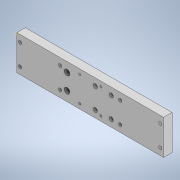
# Autodesk Inventor part: Head Adapter Plate
Saved by Autodesk Inventor 2020 (Build 240168000, 168)
## iProperties
Created: 2020-03-19
Part Number: Head Adapter Plate
Material: Generic
Document SubType Name: Modeling
Designer: DasNick
Density: 1 g/cm^3
Appearance: Default
Author: DasNick
Autodesk Inventor part; units mm, degrees
ref_plane "YZ Plane" through (0, 0, 0) normal (1, 0, 0) x (0, 1, 0)
ref_plane "XZ Plane" through (0, 0, 0) normal (0, 1, 0) x (-1, 0, 0)
ref_plane "XY Plane" through (0, 0, 0) normal (0, 0, 1) x (1, 0, 0)
sketch "Sketch1" plane through (0, 0, 0) normal (0, 0, 1) x (1, 0, 0)
  line L0 (13.4603, 15.4458) -> (13.4545, -36.9417)
  circle A0 centre (18.2181, -26.6234) radius 2.3812
  circle A1 centre (18.2217, 5.1266) radius 2.3812
  circle A2 centre (78.5467, 5.1199) radius 2.3812
  circle A3 centre (78.5431, -26.6301) radius 2.3812
  circle A4 centre (169.0306, -26.6401) radius 2.3812
  circle A5 centre (229.3556, -26.6468) radius 2.3812
  circle A6 centre (229.3592, 5.1032) radius 2.3812
  line L1 (234.1228, 15.4214) -> (234.117, -36.9661)
  circle A7 centre (169.0342, 5.1099) radius 2.3812
  line L2 (13.4545, -36.9417) -> (234.117, -36.9661)
  line L3 (234.1228, 15.4214) -> (13.4603, 15.4458)
  point P0 (3.3527, -2.3752)
  constraints: 8 centre point, 8 end point
extrude "Extrusion1" add sketch "Sketch1" along normal blind 12.7
sketch "Sketch3" plane through (0, 0, 0) normal (0, 0, -1) x (-1, 0, 0)
  line L0 (-234.117, -36.9661) -> (-234.1228, 15.4214) projected
  line L1 (-234.1199, -10.7723) -> (-13.4574, -10.7479)
  line L2 (-13.4603, 15.4458) -> (-13.4545, -36.9417) projected
  line L3 (-234.1228, 15.4214) -> (-13.4603, 15.4458) projected
  line L4 (-123.7915, 15.4336) -> (-123.7857, -36.9539)
  line L5 (-13.4545, -36.9417) -> (-234.117, -36.9661) projected
  circle A0 centre (-155.5369, -26.2636) radius 1.5
  circle A1 centre (-131.5369, -26.261) radius 1.5
  circle A2 centre (-155.5404, 4.7364) radius 1.5
  circle A3 centre (-131.5404, 4.739) radius 1.5
  point P0 (0, 0)
  dimension "d8" = 15.5
  dimension "d9" = 31.75
  dimension "d10" = 3
  dimension "d13" = 24
  dimension "d16" = 31
  constraints: 4 centre point, 4 end point, 3 midpoint, 10 other
  measures "d8" distance from line of L1 A0.centre
  measures "d9" distance from line of L4 A0.centre
  measures "d10" diameter of A0
  measures "d13" distance of A0.centre A1.centre
  measures "d16" distance of A0.centre A2.centre
extrude "Extrusion2" cut sketch "Sketch3" against normal blind 12.7 contours A0 | A1 | A2 | A3
sketch "Sketch4" plane through (0, 0, 0) normal (0, 0, -1) x (-1, 0, 0)
  circle A0 centre (-131.5369, -26.261) radius 1.5 projected
  circle A1 centre (-131.5369, -26.261) radius 3.175
  circle A2 centre (-155.5369, -26.2636) radius 1.5 projected
  circle A3 centre (-155.5369, -26.2636) radius 3.175
  circle A4 centre (-131.5404, 4.739) radius 1.5 projected
  circle A5 centre (-131.5404, 4.739) radius 3.175
  circle A6 centre (-155.5404, 4.7364) radius 1.5 projected
  circle A7 centre (-155.5404, 4.7364) radius 3.175
  point P0 (0, 0)
  dimension "d21" = 6.35
  dimension "d22" = 6.35
  dimension "d23" = 6.35
  dimension "d24" = 6.35
  constraints: 4 centre point, 4 coincident
  measures "d21" diameter of A1
  measures "d22" diameter of A3
  measures "d23" diameter of A5
  measures "d24" diameter of A7
extrude "Extrusion3" cut sketch "Sketch4" against normal blind 3.175
sketch "Sketch5" plane through (0, 0, 0) normal (0, 0, -1) x (-1, 0, 0)
  point P0 (0, 0)
sketch "Sketch6" plane through (0, 0, 0) normal (0, 0, -1) x (-1, 0, 0)
  point P0 (0, 0)
sketch "Sketch7" plane through (0, 0, 0) normal (0, 0, -1) x (-1, 0, 0)
  point P0 (0, 0)
sketch "Sketch8" plane through (0, 0, 0) normal (0, 0, -1) x (-1, 0, 0)
  circle A0 centre (-108.2333, 8.2916) radius 1.5875
  line L0 (-234.1228, 15.4214) -> (-13.4603, 15.4458) construction
  line L1 (-123.7915, 15.4336) -> (-123.7857, -36.9539) construction
  line L2 (-13.4545, -36.9417) -> (-234.117, -36.9661) construction
  line L3 (-234.117, -36.9661) -> (-234.1228, 15.4214) construction
  line L4 (-234.1199, -10.7723) -> (-13.4574, -10.7479) construction
  line L5 (-13.4603, 15.4458) -> (-13.4545, -36.9417) construction
  circle A1 centre (-108.229, -29.8084) radius 1.5875
  circle A2 centre (-139.9833, 8.2881) radius 1.5875
  circle A3 centre (-139.979, -29.8119) radius 1.5875
  point P0 (0, 0)
  dimension "d27" = 3.175
  dimension "d28" = 15.5575
  dimension "d31" = 38.1
  dimension "d34" = 31.75
  dimension "d37" = 19.05
  constraints: 4 centre point, 4 end point, 4 midpoint, 8 other
  measures "d27" diameter of A0
  measures "d28" distance from line of L1 A0.centre
  measures "d31" distance of A0.centre A1.centre
  measures "d34" distance of A0.centre A2.centre
  measures "d37" distance from line of L4 A0.centre
extrude "Extrusion4" cut sketch "Sketch8" against normal blind 25.4
sketch "Sketch9" plane through (0, 0, 12.7) normal (0, 0, 1) x (1, 0, 0)
  circle A0 centre (155.5369, -26.2636) radius 1.5 projected
  circle A1 centre (131.5369, -26.261) radius 1.5 projected
  circle A2 centre (155.5404, 4.7364) radius 1.5 projected
  circle A3 centre (131.5404, 4.739) radius 1.5 projected
  circle A4 centre (155.5369, -26.2636) radius 3.175
  circle A5 centre (131.5369, -26.261) radius 3.175
  circle A6 centre (131.5404, 4.739) radius 3.175
  circle A7 centre (155.5404, 4.7364) radius 3.175
  point P0 (0, 0)
  dimension "d40" = 6.35
  dimension "d41" = 6.35
  dimension "d42" = 6.35
  dimension "d43" = 6.35
  constraints: 4 centre point, 4 coincident
  measures "d40" diameter of A4
  measures "d41" diameter of A5
  measures "d42" diameter of A6
  measures "d43" diameter of A7
extrude "Extrusion5" cut sketch "Sketch9" against normal blind 3.175
sketch "Sketch10" plane through (0, 0, 0) normal (0, 0, -1) x (-1, 0, 0)
  circle A0 centre (-88.9984, 1.2723) radius 3.175 projected
  circle A1 centre (-88.9953, -22.4777) radius 3.175 projected
  circle A2 centre (-88.9953, -22.4777) radius 3.9688
  circle A3 centre (-88.9984, 1.2723) radius 3.9688
  point P0 (0, 0)
  dimension "d46" = 7.9375
  dimension "d47" = 7.9375
  constraints: 2 centre point, 2 coincident
  measures "d46" diameter of A2
  measures "d47" diameter of A3
extrude "Extrusion6" cut sketch "Sketch10" against normal blind 12.7 contours A0 | A1 | A2 | A3
fillet "Fillet1" radius 0.254 4 edges at (92.9672, 1.2723, 12.7) (92.9641, -22.4777, 12.7) (92.9641, -22.4777, 0) (92.9672, 1.2723, 0)
sketch "Sketch11" plane through (0, 0, 0) normal (0, 0, -1) x (-1, 0, 0)
  circle A0 centre (-88.9953, -22.4777) radius 3.9688
  circle A1 centre (-139.979, -29.8119) radius 1.5875
  circle A2 centre (-139.9833, 8.2881) radius 1.5875
  circle A3 centre (-108.229, -29.8084) radius 1.5875
  circle A4 centre (-108.2333, 8.2916) radius 1.5875
  circle A5 centre (-155.5404, 4.7364) radius 3.175
  circle A6 centre (-155.5369, -26.2636) radius 3.175
  circle A7 centre (-131.5404, 4.739) radius 3.175
  circle A8 centre (-131.5369, -26.261) radius 3.175
  line L0 (-13.4545, -36.9417) -> (-234.117, -36.9661)
  line L1 (-13.4603, 15.4458) -> (-13.4545, -36.9417)
  line L2 (-234.1228, 15.4214) -> (-13.4603, 15.4458)
  line L3 (-234.117, -36.9661) -> (-234.1228, 15.4214)
  circle A9 centre (-169.0342, 5.1099) radius 2.3812
  circle A10 centre (-229.3592, 5.1032) radius 2.3812
  circle A11 centre (-229.3556, -26.6468) radius 2.3812
  circle A12 centre (-169.0306, -26.6401) radius 2.3812
  circle A13 centre (-78.5431, -26.6301) radius 2.3812
  circle A14 centre (-78.5467, 5.1199) radius 2.3812
  circle A15 centre (-18.2217, 5.1266) radius 2.3812
  circle A16 centre (-18.2181, -26.6234) radius 2.3812
  circle A17 centre (-88.9984, 1.2723) radius 4.2227
  point P0 (0, 0)
  dimension "d51" = 10.3187
  dimension "d53" = 4.7625
  dimension "d54" = 220.6625
  dimension "d55" = 4.7625
  dimension "d56" = 65.0875
  dimension "d57" = 94.7738
  dimension "d58" = 118.0812
  dimension "d59" = 7.9375
  dimension "d60" = 126.5238
  dimension "d61" = 142.0813
  dimension "d62" = 155.575
  dimension "d63" = 215.9
  dimension "d64" = 14.4724
  dimension "d65" = 42.0688
  dimension "d66" = 7.1437
  dimension "d67" = 38.2224
  dimension "d68" = 10.6937
  dimension "d69" = 45.2437
  dimension "d70" = 41.6938
  dimension "d71" = 52.3875
  constraints: 35 centre point, 8 end point
  measures "d51" distance from line of L0 A16.centre
  measures "d53" diameter of A16
  measures "d54" distance of L0.start L0.end
  measures "d55" distance from line of A16.centre L1
  measures "d56" distance from line of A13.centre L1
  measures "d57" distance from line of A3.centre L1
  measures "d58" distance from line of A8.centre L1
  measures "d59" diameter of A0
  measures "d60" distance from line of L1 A1.centre
  measures "d61" distance from line of L1 A6.centre
  measures "d62" distance from line of L1 A12.centre
  measures "d63" distance from line of L1 A11.centre
  measures "d64" distance from line of L0 A0.centre
  measures "d65" distance from line of A15.centre L0
  measures "d66" distance from line of L0 A3.centre
  measures "d67" distance from line of A17.centre L0
  measures "d68" distance from line of A8.centre L0
  measures "d69" distance from line of A4.centre L0
  measures "d70" distance from line of A5.centre L0
  measures "d71" distance of L0.end L2.start
body "Solid1"
